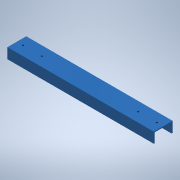
# Autodesk Inventor part: ADSK-MH-10011
Saved by Autodesk Inventor 2020.2 (Build 242310000, 310)
## iProperties
Created: 2008-03-10
Part Number: ADSK-MH-10011
Document SubType Name: Modeling
Designer: R.O'mahony
Density: 7.86 g/cm^3
Mass: 745.702 g
Surface Area: 3107.39 cm^2
Volume: 745.702 cm^3
Material: Steel, Mild
Appearance: Cyan
Description: Top Support
Engineer: Demir Ali
Checked By: Demir Ali
Company: Autodesk Ltd
Author: R.O'mahony
Keywords: Roller Conveyor
Revision Number: A
Autodesk Inventor part; units mm, degrees
ref_plane "YZ Plane" through (0, 0, 0) normal (1, 0, 0) x (0, 1, 0)
ref_plane "XZ Plane" through (0, 0, 0) normal (0, 1, 0) x (-1, 0, 0)
ref_plane "XY Plane" through (0, 0, 0) normal (0, 0, 1) x (1, 0, 0)
sketch "Sketch1" plane through (0, 0, 0) normal (0, 0, 1) x (1, 0, 0)
  line L0 (-350, 45) -> (350, 45)
  line L1 (-350, -45) -> (350, -45)
  line L2 (-350, 45) -> (-350, -45)
  line L3 (350, 45) -> (350, -45)
  line L4 (350, -45) -> (-350, 45) construction
  line L5 (-350, -45) -> (350, 45) construction
  point P0 (0, 0)
  point P1 (0, 0)
  dimension "d8" = 700
  dimension "d9" = 90
  constraints: 12 end point, 2 parallel, 1 coincident, 1 horizontal, 1 midpoint, 1 perpendicular
  measures "d8" distance of L0.start L0.end
  measures "d9" distance of L0.start L1.start
extrude "Extrusion1" add sketch "Sketch1" against normal blind 50
shell "Shell1" thickness 5 removed faces 3 at (350, 15, -16.6667) at (-350, -15, -16.6667) at (116.6667, 15, -50)
sketch "Sketch3" plane through (0, 0, 0) normal (0, 0, 1) x (1, 0, 0)
  point P0 (0, 0)
  point P1 (320, 0)
  point P2 (230, 0)
  dimension "d11" = 320
  dimension "d12" = 90
  constraints: 2 horizontal alignment
  measures "d11" distance of point (320, 0) point (0, 0)
  measures "d12" distance of point (320, 0) point (230, 0)
hole "Hole1" at (320, 0, 0) at (230, 0, 0) direction (0, 0, -1) diameter 8.376 end through all thread size "M10x1.5" class "6H" standard "ANSI Metric M Profile"
pattern_circular "Circular Pattern1" count 2 over 360 about axis through (0, 0, -10) along (0, 0, 1) of "Hole1"
body "Solid1"
